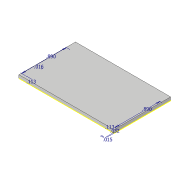
# Autodesk Inventor part: Sharp 2Y0A02 Case Lid
Saved by Autodesk Inventor 2018.3 (Build 223284000, 284)
## iProperties
Created: 2018-12-13
Part Number: Sharp 2Y0A02 Case Lid
Material: Generic
Document SubType Name: Modeling
Designer: aye06091
Mass: 2.17423 g
Surface Area: 29.8209 cm^2
Volume: 2.17423 cm^3
Density: 1 g/cm^3
Appearance: Default
Author: aye06091
Autodesk Inventor part; units mm, degrees
ref_plane "YZ Plane" through (0, 0, 0) normal (1, 0, 0) x (0, 1, 0)
ref_plane "XZ Plane" through (0, 0, 0) normal (0, 1, 0) x (-1, 0, 0)
ref_plane "XY Plane" through (0, 0, 0) normal (0, 0, 1) x (1, 0, 0)
sketch "Sketch1" plane through (0, 0, 0) normal (0, 1, 0) x (-1, 0, 0)
  line L0 (0, 0) -> (-47.9298, 0)
  line L1 (-47.9298, 0) -> (-47.9298, 28.575)
  line L2 (-47.9298, 28.575) -> (0, 28.575)
  line L3 (0, 28.575) -> (0, 0)
  dimension "d0" = 47.9298
  dimension "d1" = 28.575
  constraints: 8 end point, 2 parallel, 1 horizontal, 1 perpendicular
  measures "d0" distance of L0.start L0.end
  measures "d1" distance of L2.end L0.start
extrude "Extrusion1" add sketch "Sketch1" along normal blind 1.5875
sketch "Sketch2" plane through (0, 0, 0) normal (0, -1, 0) x (1, 0, 0)
  line L0 (0, 0) -> (47.9298, 0) projected
  line L1 (47.9298, 0) -> (47.9298, 28.575) projected
  line L2 (47.9298, 28.575) -> (0, 28.575) projected
  line L3 (0, 28.575) -> (0, 0) projected
  line L4 (47.5456, 3.1115) -> (46.7265, 3.1115)
  line L5 (46.7265, 3.1115) -> (46.7265, 25.7175)
  line L6 (46.7265, 25.7175) -> (47.5456, 25.7175)
  line L7 (47.5456, 25.7175) -> (47.5456, 3.1115)
  line L8 (1.8398, 25.7175) -> (0.3969, 25.7175)
  line L9 (0.3969, 25.7175) -> (0.3969, 3.1115)
  line L10 (0.3969, 3.1115) -> (1.8398, 3.1115)
  line L11 (1.8398, 3.1115) -> (1.8398, 25.7175)
  dimension "d4" = 22.606
  dimension "d5" = 22.606
  dimension "d6" = 2.8575
  dimension "d7" = 2.8575
  dimension "d8" = 0.3842
  dimension "d9" = 0.3969
  dimension "d10" = 0.8192
  constraints: 16 end point, 4 parallel, 2 horizontal, 2 perpendicular
  measures "d4" distance of L4.end L5.end
  measures "d5" distance of L8.end L9.end
  measures "d6" distance between parallel lines of L2 L6
  measures "d7" distance between parallel lines of L2 L8
  measures "d8" distance between parallel lines of L1 L7
  measures "d9" distance between parallel lines of L3 L9
  measures "d10" distance of L5.end L6.end
body "Solid1"
